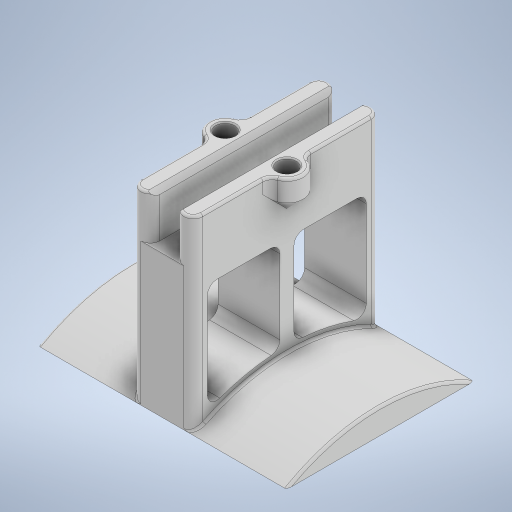
# Autodesk Inventor part: FuselageMount
Saved by Autodesk Inventor 2023 (Build 270158000, 158)
## iProperties
Created: 2023-11-15
Part Number: FuselageMount
Material: Generic
Document SubType Name: Modeling
Designer: Eric
Density: 1 g/cm^3
Appearance: Default
Author: Eric
Autodesk Inventor part; units mm, degrees
ref_plane "YZ Plane" through (0, 0, 0) normal (1, 0, 0) x (0, 1, 0)
ref_plane "XZ Plane" through (0, 0, 0) normal (0, 1, 0) x (-1, 0, 0)
sketch "Sketch1" plane through (0, 0, 0) normal (1, 0, 0) x (0, 1, 0)
  line L0 (0, 0) -> (40, 0)
  line L1 (40, 0) -> (40, -40)
  line L2 (40, -40) -> (0, -40)
  line L3 (0, -40) -> (0, 0)
  dimension "d0" = 40
  dimension "d1" = 40
  constraints: 8 end point, 2 parallel, 1 horizontal, 1 perpendicular
  measures "d0" distance of L0.start L0.end
  measures "d1" distance of L2.end L0.start
extrude "Extrusion1" add sketch "Sketch1" along normal blind 13.2
sketch "Sketch2" plane through (13.2, 0, 0) normal (1, 0, 0) x (0, 0, -1)
  line L0 (40, 0) -> (40, 40) projected
  line L1 (0, 40) -> (0, 0) projected
  line L2 (0, 0) -> (40, 0) projected
  line L3 (0, 0) -> (40, 0)
  arc A0 (40, 0) -> (0, 0) centre (20, -34.641) ccw
  dimension "d30" = 40
  constraints: 2 end point, 2 point on circle, 1 centre point, 1 collinear
  measures "d30" radius of A0
extrude "Extrusion2" add sketch "Sketch2" along normal blind 20
ref_plane "Work Plane1" through (6.6, 0, 0) normal (-1, 0, 0) x (0, 0, 1)
mirror "Mirror1" about plane through (6.6, 0, 0) normal (-1, 0, 0) of "Extrusion2"
sketch "Sketch3" plane through (0, 40, 0) normal (0, 1, 0) x (1, 0, 0)
  line L0 (0, 40) -> (13.2, 40) projected
  line L1 (0, 0) -> (13.2, 0) projected
  line L2 (4, 40) -> (9.2, 40)
  line L3 (9.2, 40) -> (9.2, 0)
  line L4 (9.2, 0) -> (4, 0)
  line L5 (4, 0) -> (4, 40)
  line L6 (0, 40) -> (0, 0) projected
  dimension "d8" = 5.2
  dimension "d9" = 4
  constraints: 8 end point, 2 parallel, 2 point on line, 1 horizontal, 1 perpendicular
  measures "d8" distance between parallel lines of L3 L5
  measures "d9" distance between parallel lines of L6 L5
extrude "Extrusion3" cut sketch "Sketch3" against normal blind 9.6 contours L0 L3 L1 L5
sketch "Sketch4" plane through (13.2, 40, 0) normal (0, 1, 0) x (1, 0, 0)
  circle A0 centre (0, 20) radius 2.05
  line L0 (-13.2, 40) -> (-13.2, 0) projected
  circle A1 centre (-13.2, 20) radius 2.05
  circle A2 centre (0, 20) radius 3.5
  circle A3 centre (-13.2, 20) radius 3.5
  line L1 (0, 40) -> (0, 0) projected
  dimension "d16" = 4.1
  dimension "d17" = 7
  constraints: 4 centre point, 2 coincident, 2 equal radius, 2 midpoint
  measures "d16" diameter of A0
  measures "d17" diameter of A2
extrude "Extrusion4" add sketch "Sketch4" against normal blind 8
extrude "Extrusion5" cut sketch "Sketch4" against normal blind 3.1 contours A0 L1 | L1 A0 | A1 L0 | L0 A1
sketch "Sketch5" plane through (13.2, 0, 0) normal (1, 0, 0) x (0, 0, -1)
  line L0 (3, 26.4) -> (37, 26.4)
  line L1 (37, 26.4) -> (37, 3)
  line L2 (3, 26.4) -> (3, 3)
  arc A0 (37, 3) -> (3, 3) centre (20, -35.4057) ccw
  line L3 (0, 40) -> (0, 0) projected
  line L4 (40, 0) -> (40, 40) projected
  line L5 (0, 0) -> (40, 0) projected
  line L6 (18.5, 26.4) -> (18.5, 6.5675)
  line L7 (21.5, 26.4) -> (21.5, 6.5675)
  point P0 (0, 30.4)
  point P1 (20, 0)
  dimension "d31" = 3
  dimension "d32" = 3
  dimension "d33" = 4
  dimension "d34" = 3
  dimension "d35" = 42
  dimension "d39" = 3
  dimension "d40" = 1.5
  constraints: 10 end point, 4 point on circle, 2 parallel, 2 point on line, 1 centre point, 1 horizontal, 1 horizontal alignment, 1 midpoint, 1 perpendicular, 1 vertical
  measures "d31" distance between parallel lines of L3 L2
  measures "d32" distance between parallel lines of L4 L1
  measures "d33" distance from line of point (0, 30.4) L0
  measures "d34" distance from line of L5 L2.end
  measures "d35" radius of A0
  measures "d39" distance between parallel lines of L6 L7
  measures "d40" distance from line of point (20, 0) L6
extrude "Extrusion6" cut sketch "Sketch5" against normal up to surface (13.2 mm away) contours L0 L6 A0 L2 | L0 L1 A0 L7
chamfer "Chamfer2" distance 3.5 angle 45 2 edges at (-3.5, 32, -20) (16.7, 32, -20)
fillet "Fillet1" radius 2 8 edges at (0, 20, -40) (4, 35.2, -40) (9.2, 35.2, -40) (13.2, 20, -40) (13.2, 20, 0) (9.2, 35.2, 0) (4, 35.2, 0) (0, 20, 0)
chamfer "Chamfer1" distance 1 angle 45 2 edges at (9.2, 40, -20) (4, 40, -20)
fillet "Fillet2" radius 2 4 edges at (0, 37.7499, -23.5) (0, 37.7499, -16.5) (13.2, 37.7499, -23.5) (13.2, 37.7499, -16.5)
fillet "Fillet3" radius 0.5 22 edges at (-0.3486, 40, -23.9953) (-0.3486, 40, -16.0047) (-3.5, 40, -20) (0, 40, -31.5617) (0, 40, -8.4383) (1, 40, -39.7321) (1, 40, -0.2679) (13.5486, 40, -16.0047) (13.5486, 40, -23.9953) (16.7, 40, -20) (13.2, 40, -31.5617) (13.2, 40, -8.4383) (12.2, 40, -39.7321) (12.2, 40, -0.2679) (0.6289, 0.3084, -0.5439) (0.6272, 0.3093, -39.4544) (0, 5.359, -20) (-20, 5.359, -20) (12.5728, 0.3093, -39.4545) (12.5711, 0.3084, -0.5439) (13.2, 5.359, -20) (33.2, 5.359, -20)
chamfer "Chamfer3" distance 0.25 angle 45 2 edges at (-2.05, 40, -20) (11.15, 40, -20)
fillet "Fillet4" radius 2 8 edges at (6.6, 3, -37) (6.6, 3, -3) (6.6, 26.4, -37) (6.6, 26.4, -3) (6.6, 26.4, -18.5) (6.6, 26.4, -21.5) (6.6, 6.5675, -21.5) (6.6, 6.5675, -18.5)
body "Solid1"
